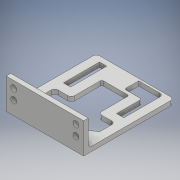
# Autodesk Inventor part: OpenMVMount-Tate
Saved by Autodesk Inventor 2018 (Build 220112000, 112)
## iProperties
Created: 2018-11-18
Part Number: OpenMVMount-Tate
Material: 一般
Document SubType Name: Modeling
Designer: shun2
Density: 1 g/cm^3
Appearance: 既定
Author: shun2
Autodesk Inventor part; units mm, degrees
ref_plane "YZ Plane" through (0, 0, 0) normal (1, 0, 0) x (0, 1, 0)
ref_plane "XZ Plane" through (0, 0, 0) normal (0, 1, 0) x (-1, 0, 0)
ref_plane "XY Plane" through (0, 0, 0) normal (0, 0, 1) x (1, 0, 0)
sketch "スケッチ1" plane through (0, 0, 0) normal (0, 0, 1) x (1, 0, 0)
  arc A0 (-12.1121, -20.6138) -> (-14.0201, -20.6138) centre (-13.0661, -20.6138) ccw
  arc A1 (-14.0201, -20.6138) -> (-12.1121, -20.6138) centre (-13.0661, -20.6138) ccw
  arc A2 (14.9359, -20.6138) -> (16.8439, -20.6138) centre (15.8899, -20.6138) ccw
  arc A3 (16.8439, -20.6138) -> (14.9359, -20.6138) centre (15.8899, -20.6138) ccw
  arc A4 (-8.2902, -23.9158) -> (-16.3681, -15.2115) centre (-21.4196, -28) ccw
  arc A5 (19.2289, -15.2115) -> (11.1509, -23.9158) centre (24.2804, -28) ccw
  line L0 (4.7797, 20.581) -> (4.7797, 15.1081)
  line L1 (5.7797, 14.1081) -> (13.9359, 14.1081)
  line L2 (14.9359, 13.1081) -> (14.9359, -0.6888)
  line L3 (-12.1121, 20.581) -> (-12.1121, -0.6888)
  line L4 (-16.3681, -15.2115) -> (-16.3681, -7.8183)
  line L5 (-16.3681, -0.6888) -> (-16.3681, 20.581)
  line L6 (-16.3681, -0.6888) -> (-12.1121, -0.6888)
  line L7 (14.9359, -0.6888) -> (19.2289, -0.6888)
  line L8 (19.2289, -15.2115) -> (19.2289, -7.8183)
  line L9 (19.2289, -0.6888) -> (19.2289, 20.581)
  line L10 (-14.3681, -5.8183) -> (-8.6023, -5.8183)
  line L11 (11.461, -5.8183) -> (17.2289, -5.8183)
  line L12 (-16.3681, 20.581) -> (-12.1121, 20.581)
  line L13 (4.7797, 20.581) -> (4.7797, 22.581)
  line L14 (4.7797, 22.581) -> (17.2289, 22.581)
  line L15 (19.2289, 20.581) -> (19.2289, 20.581)
  arc A6 (-8.6023, -5.8183) -> (-6.6023, -3.8183) centre (-8.6023, -3.8183) ccw
  arc A7 (9.461, -3.8183) -> (11.461, -5.8183) centre (11.461, -3.8183) ccw
  arc A8 (-14.3681, -5.8183) -> (-16.3681, -7.8183) centre (-14.3681, -7.8183) ccw
  arc A9 (19.2289, -7.8183) -> (17.2289, -5.8183) centre (17.2289, -7.8183) ccw
  arc A10 (19.2289, 20.581) -> (17.2289, 22.581) centre (17.2289, 20.581) ccw
  line L16 (-21.4196, 23.7891) -> (-21.4196, -23.9158)
  line L17 (24.2059, 23.7891) -> (-21.4196, 23.7891)
  line L18 (9.461, -3.8183) -> (9.461, 11.1956)
  line L19 (8.461, 12.1956) -> (-5.6023, 12.1956)
  line L20 (-6.6023, 11.1956) -> (-6.6023, -3.8183)
  line L21 (24.2059, -23.9158) -> (24.2059, 23.7891)
  arc A11 (14.9359, 13.1081) -> (13.9359, 14.1081) centre (13.9359, 13.1081) ccw
  arc A12 (4.7797, 15.1081) -> (5.7797, 14.1081) centre (5.7797, 15.1081) ccw
  arc A13 (9.461, 11.1956) -> (8.461, 12.1956) centre (8.461, 11.1956) ccw
  arc A14 (-5.6023, 12.1956) -> (-6.6023, 11.1956) centre (-5.6023, 11.1956) ccw
  line L22 (24.2059, -23.9158) -> (24.2059, -26.6158)
  line L23 (24.2059, -26.6158) -> (-21.4196, -26.6158)
  line L24 (-21.4196, -26.6158) -> (-21.4196, -23.9158)
  line L25 (-8.2902, -23.9158) -> (11.1509, -23.9158)
  point P0 (0, 0)
  point P1 (8.6618, 1.6271)
  point P2 (12.2118, 1.6271)
  dimension "d0" = 27.5
  dimension "d1" = 27.5
  dimension "d2" = 2
  dimension "d5" = 1
  dimension "d6" = 2.7
  constraints: 52 end point, 31 point on circle, 16 tangent, 15 centre point, 12 perpendicular, 6 equal radius, 6 vertical, 3 horizontal, 2 parallel
  measures "d0" diameter of A4
  measures "d1" diameter of A5
  measures "d2" radius of A6
  measures "d5" radius of A11
  measures "d6" distance of L21.start L23.start
extrude "押し出し1" add sketch "スケッチ1" along normal blind 2.7
sketch "スケッチ2" plane through (0, 0, 0) normal (0, 0, -1) x (-1, 0, 0)
  line L0 (21.4196, -26.6158) -> (-24.2059, -26.6158) projected
  line L1 (21.4196, -26.6158) -> (-24.2059, -26.6158)
  line L2 (-24.2059, -26.6158) -> (-24.2059, -29.3158)
  line L3 (-24.2059, -29.3158) -> (21.4196, -29.3158)
  line L4 (21.4196, -29.3158) -> (21.4196, -26.6158)
  point P0 (0, 0)
  dimension "d9" = 2.7
  constraints: 8 end point, 2 parallel, 1 horizontal, 1 perpendicular
  measures "d9" distance of L2.end L1.end
extrude "押し出し2" add sketch "スケッチ2" against normal blind 18
sketch "スケッチ3" plane through (-21.4196, -26.6158, 2.7) normal (0, 1, 0) x (1, 0, 0)
  circle A0 centre (4.5, -11.3) radius 1.75
  line L0 (45.6256, -15.3) -> (0, -15.3) projected
  line L1 (0, 0) -> (0, -15.3) projected
  circle A1 centre (4.5, -5.3) radius 1.75
  circle A2 centre (41.1256, -11.3) radius 1.75
  line L2 (45.6256, 0) -> (45.6256, -15.3) projected
  circle A3 centre (41.1256, -5.3) radius 1.75
  point P0 (21.4196, 2.7)
  dimension "d12" = 3.5
  dimension "d13" = 4
  dimension "d14" = 4.5
  dimension "d15" = 3.5
  dimension "d16" = 3.5
  dimension "d17" = 10
  dimension "d18" = 4.5
  dimension "d19" = 3.5
  constraints: 4 centre point
  measures "d12" diameter of A0
  measures "d13" distance from line of L0 A0.centre
  measures "d14" distance from line of L1 A0.centre
  measures "d15" diameter of A1
  measures "d16" diameter of A2
  measures "d17" distance from line of L0 A1.centre
  measures "d18" distance from line of L2 A2.centre
  measures "d19" diameter of A3
extrude "押し出し3" cut sketch "スケッチ3" against normal blind 2.7
fillet "フィレット1" radius 2 2 edges at (-21.4196, 23.7891, 1.35) (24.2059, 23.7891, 1.35)
chamfer "面取り1" distance 1.3 angle 45 1 edges at (1.3931, -26.6158, 2.7)
